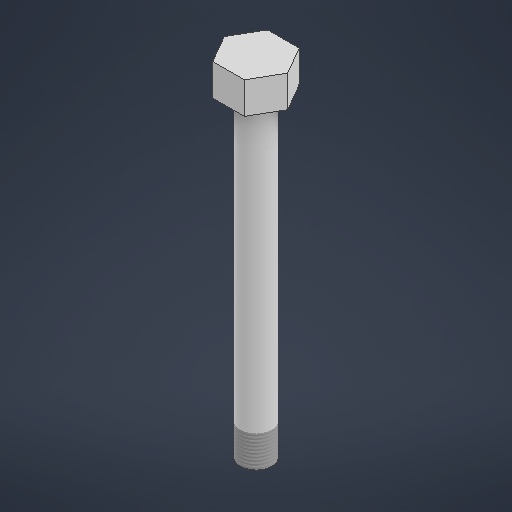
# Autodesk Inventor part: BoltA
Saved by Autodesk Inventor 2026.1 (Build 301233020, 233B)
## iProperties
Created: 2025-11-04
Part Number: BoltA
Material: Generic
Document SubType Name: Modeling
Designer: Study
Density: 1 g/cm^3
Appearance: Default
Author: Study
Autodesk Inventor part; units mm, degrees
ref_plane "YZ Plane" through (0, 0, 0) normal (1, 0, 0) x (0, 1, 0)
ref_plane "XZ Plane" through (0, 0, 0) normal (0, 1, 0) x (-1, 0, 0)
ref_plane "XY Plane" through (0, 0, 0) normal (0, 0, 1) x (1, 0, 0)
sketch "Sketch1" plane through (0, 0, 0) normal (0, 1, 0) x (-1, 0, 0)
  circle A0 centre (0, 0) radius 5
  dimension "d0" = 10
  constraints: 1 centre point, 1 coincident
  measures "d0" diameter of A0
extrude "Extrusion1" add sketch "Sketch1" along normal blind 100
thread "Thread1" size "M10x1" class "6g" standard "ISO Metric profile" length 10
sketch "Sketch2" plane through (0, 100, 0) normal (0, 1, 0) x (1, 0, 0)
  circle A0 centre (0, 0) radius 5 projected
  circle A1 centre (0, 0) radius 10 construction
  line L0 (-10, 0) -> (-5, 8.6603)
  line L1 (-5, 8.6603) -> (5, 8.6603)
  line L2 (5, 8.6603) -> (10, 0)
  line L3 (10, 0) -> (5, -8.6603)
  line L4 (5, -8.6603) -> (-5, -8.6603)
  line L5 (-5, -8.6603) -> (-10, 0)
  dimension "d5" = 20
  constraints: 12 end point, 2 coincident, 1 horizontal alignment, 15 other
extrude "Extrusion2" add sketch "Sketch2" along normal blind 10 contours A0 | L0 L1 L2 L3 L4 L5
body "Solid1"
